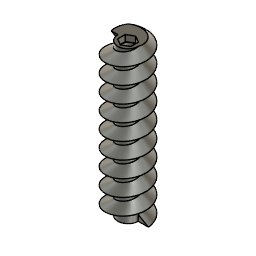
Archimedes_Screw (Autodesk Fusion 360 design; units mm, degrees)
Autodesk Fusion 360 part; units mm, degrees
note: some values were not read from the file. Chosen so that the rebuilt part matches the saved one: which bodies a step acts on.
cylinder "Grundkörper Zylinder1" add diameter 20 height 148 placed x (1, 0, 0) y (0, 1, 0) z (0, 0, 1) at (0, 0, 0) makes body 1
cylinder "Grundkörper Zylinder2" cut diameter 12.8 height -148 placed x (1, 0, 0) y (0, 1, 0) z (0, 0, 1) at (0, 0, 148) bodies 1
coil "Grundkörper Spirale1" add diameter 30 section triangle out size 10 on centre turns 9.5 pitch 15.78947 right hand placed x (1, 0, 0) y (0, 1, 0) z (0, 0, 1) at (0, 0, 0) separate body makes body 2
split "Teilen1" by plane through (0, 0, 148) normal (0, 0, 1) and through (0, 0, 0) normal (0, 0, -1) bodies 2 makes body 3 at (16.4555, 0.7364, -1.9245) makes body 4 at (-11.8461, 11.5872, 150.0339)
delete_body "Körper entfernen1" bodies 3
delete_body "Körper entfernen2" bodies 4
combine "Kombinieren1" operation add target body 2 tool bodies 1
sketch "Skizze6" plane through (0, 0, 0) normal (0, 0, 1) x (1, 0, 0)
  line L0 (6.45, 3.7239) -> (0, 7.4478)
  line L1 (0, 7.4478) -> (-6.45, 3.7239)
  line L2 (-6.45, 3.7239) -> (-6.45, -3.7239)
  line L3 (-6.45, -3.7239) -> (0, -7.4478)
  line L4 (0, -7.4478) -> (6.45, -3.7239)
  line L5 (6.45, -3.7239) -> (6.45, 3.7239)
  dimension "d13" = 6.45
  measures "d13" distance of origin L5
extrude "Extrusion1" add sketch "Skizze6" along normal blind 6 separate body makes body 5
ref_plane "Arbeitsebene1" through (-3.2696, 2.8457, 74) normal (0, 0, 1) x (1, 0, 0)
mirror "Spiegeln1" about plane through (-3.2696, 2.8457, 74) normal (0, 0, 1) of bodies 5 makes body 6
combine "Kombinieren2" operation cut target body 2 tool bodies 5 6
named bodies: "Archimedes Screw"
